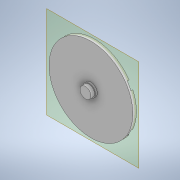
# Autodesk Inventor part: plato
Saved by Autodesk Inventor 2020 (Build 240168000, 168)
## iProperties
Created: 2019-09-28
Part Number: plato
Material: Genérico
Document SubType Name: Modeling
Designer: Java9
Density: 1 g/cm^3
Appearance: Valor por defecto
Author: Java9
Autodesk Inventor part; units mm, degrees
ref_plane "YZ Plane" through (0, 0, 0) normal (1, 0, 0) x (0, 1, 0)
ref_plane "XZ Plane" through (0, 0, 0) normal (0, 1, 0) x (-1, 0, 0)
ref_plane "XY Plane" through (0, 0, 0) normal (0, 0, 1) x (1, 0, 0)
sketch "Boceto1" plane through (0, 0, 0) normal (0, 0, 1) x (1, 0, 0)
  circle A0 centre (0, 0) radius 115
  line L0 (105, 0) -> (105, 65)
  line L1 (105, 65) -> (105, -65)
  line L2 (105, -65) -> (85, -65)
  line L3 (85, -65) -> (85, 65)
  line L4 (85, 65) -> (105, 65)
  line L5 (-105, 0) -> (-105, 65)
  line L6 (-105, 65) -> (-85, 65)
  line L7 (-85, 65) -> (-85, -65)
  line L8 (-85, -65) -> (-105, -65)
  line L9 (-105, -65) -> (-105, 0)
  dimension "d0" = 230
  dimension "d33" = 65
  dimension "d34" = 130
  dimension "d35" = 20
  dimension "d36" = 65
  dimension "d37" = 20
  constraints: 20 end point, 6 perpendicular, 2 point on line, 2 vertical, 1 centre point, 1 coincident, 1 collinear
  measures "d0" diameter of A0
  measures "d33" distance of L0.start L0.end
  measures "d34" distance of L0.end L1.end
  measures "d35" distance of L1.end L2.end
  measures "d36" distance of L5.start L5.end
  measures "d37" distance of L5.end L6.end
extrude "Extrusión1" add sketch "Boceto1" along normal blind 10 contours A0 L1 L0 | L0 L1 A0 L2 L3 L4 | L4 L3 L2 A0 L8 L7 L6 | L6 L7 L8 A0 L9 L5 | L5 L9 A0
sketch "Boceto2" plane through (0, 0, 10) normal (0, 0, 1) x (1, 0, 0)
  circle A0 centre (0, 0) radius 17.5
  circle A1 centre (0, 0) radius 14.9
  dimension "d4" = 35
  dimension "d21" = 29.8
  constraints: 3 coincident, 2 centre point
  measures "d4" diameter of A0
  measures "d21" diameter of A1
extrude "Extrusión2" add sketch "Boceto2" along normal blind 5 contours A0 | A1
sketch "Boceto3" plane through (0, 0, 15) normal (0, 0, 1) x (1, 0, 0)
  circle A0 centre (0, 0) radius 14.9
  dimension "d20" = 29.8
  constraints: 1 centre point, 1 coincident
  measures "d20" diameter of A0
extrude "Extrusión3" [suppressed]
sketch "Boceto4" plane through (0, 0, 0) normal (0, 0, -1) x (-1, 0, 0)
  line L0 (105, 0) -> (-105, 0)
  line L1 (-105, 0) -> (-105, 65)
  line L2 (-105, 65) -> (-85, 65)
  line L3 (-85, 65) -> (-85, -65)
  line L4 (-85, -65) -> (-105, -65)
  line L5 (-105, -65) -> (-105, 0)
  line L6 (105, 0) -> (105, -65)
  line L7 (105, -65) -> (85, -65)
  line L8 (85, -65) -> (85, 65)
  line L9 (85, 65) -> (105, 65)
  line L10 (105, 65) -> (105, 0)
  point P0 (0, 0)
  dimension "d40" = 65
  dimension "d41" = 20
  dimension "d42" = 130
  dimension "d43" = 65
  dimension "d44" = 20
  dimension "d45" = 130
  constraints: 22 end point, 8 perpendicular, 2 point on line, 2 vertical
  measures "d40" distance of L0.end L1.end
  measures "d41" distance of L1.end L2.end
  measures "d42" distance of L2.end L3.end
  measures "d43" distance of L0.start L6.end
  measures "d44" distance of L6.end L7.end
  measures "d45" distance of L7.end L8.end
sketch "Boceto5" plane through (0, 0, 15) normal (0, 0, 1) x (1, 0, 0)
  circle A0 centre (0, 0) radius 14.9
  dimension "d22" = 29.8
  constraints: 1 centre point, 1 coincident
  measures "d22" diameter of A0
extrude "Extrusión4" add sketch "Boceto5" along normal blind 10
ref_plane "Plano de trabajo2" through (0, 0, 5) normal (0, 0, -1) x (-1, 0, 0)
extrude "Extrusión5" cut sketch "Boceto4" against normal blind 5
